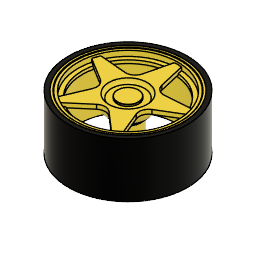
Roda (Autodesk Fusion 360 design; units mm, degrees)
part number: 2026-05-12-10-28-13-651
Autodesk Fusion 360 part; units mm, degrees
sketch "Sketch1" plane through (0, 0, 0) normal (0, 1, 0) x (1, 0, 0)
  circle A0 centre (0, 0) radius 9
  circle A1 centre (0, 0) radius 7.75
  circle A2 centre (0, 0) radius 5
  line L0 (-12.455, -19.928) -> (-2.9617, -11.8295)
  line L1 (12.3158, -20.0143) -> (2.9074, -11.8536)
  arc A3 (2.9074, -11.8536) -> (-2.9617, -11.8295) centre (-0.0412, -15.253) ccw
  line L2 (22.8405, 5.5282) -> (12.1719, -0.8978)
  arc A4 (12.1719, -0.8978) -> (10.3353, -6.4722) centre (14.4937, -4.7526) ccw
  line L3 (15.1038, -18.0035) -> (10.3353, -6.4722)
  line L4 (1.8005, 23.4309) -> (4.6152, 11.2987)
  arc A5 (4.6152, 11.2987) -> (9.3492, 7.8294) centre (8.9988, 12.3157) ccw
  line L5 (21.7896, 8.8012) -> (9.3492, 7.8294)
  line L6 (-21.7278, 8.9529) -> (-9.3195, 7.8808)
  arc A6 (-9.3195, 7.8808) -> (-4.5571, 11.3111) centre (-8.9322, 12.3641) ccw
  line L7 (-1.6371, 23.4429) -> (-4.5571, 11.3111)
  line L8 (-15.229, -17.8977) -> (-10.375, -6.4281)
  arc A7 (-10.375, -6.4281) -> (-12.1657, -0.8388) centre (-14.5192, -4.6743) ccw
  line L9 (-22.8014, 5.6873) -> (-12.1657, -0.8388)
  circle A8 centre (0, 0) radius 25
  circle A9 centre (0, 0) radius 26
  circle A10 centre (0, 0) radius 5.5
  circle A11 centre (0, 0) radius 10.5
  circle A12 centre (0, 0) radius 23.5
  circle A13 centre (0, 0) radius 21.5
  circle A14 centre (0, 0) radius 6.5
  circle A15 centre (0, 0) radius 7
  line L10 (-0.0051, -23.5) -> (-0.0226, -10.753)
  line L11 (22.3482, -7.2668) -> (10.2197, -3.3444)
  line L12 (13.8171, 19.0089) -> (6.3388, 8.6861)
  line L13 (-13.8088, 19.0149) -> (-6.3021, 8.7127)
  line L14 (-22.3514, -7.257) -> (-10.2337, -3.3013)
  circle A16 centre (0, 0) radius 2.9
  line L15 (-2.9, -1.8) -> (2.9, -1.8)
  line L16 (2.9, -1.8) -> (2.9, 1.8)
  line L17 (2.9, 1.8) -> (-2.9, 1.8)
  line L18 (-2.9, 1.8) -> (-2.9, -1.8)
  line L19 (-2.9, -1.8) -> (2.9, 1.8) construction
  line L20 (2.9, -1.8) -> (-2.9, 1.8) construction
  dimension "d7" = 18
  dimension "d8" = 15.5
  dimension "d9" = 10
  dimension "d13" = 4.5
  dimension "d15" = 360
  dimension "d16" = 50
  dimension "d17" = 52
  dimension "d18" = 11
  dimension "d19" = 21
  dimension "d20" = 47
  dimension "d35" = 43
  dimension "d48" = 13
  dimension "d67" = 14
  dimension "d83" = 360
  dimension "d98" = 5.8
  constraint coincident A0.centre A1.centre
  constraint tangent L0 A3
  constraint tangent L1 A3
  constraint concentric A0 A9
  constraint concentric A1 A10
  constraint concentric A1 A11
  constraint concentric A2 A12
  constraint coincident L9.start A12
  constraint coincident L6.start A12
  constraint concentric A2 A13
  constraint concentric A0 A14
  constraint concentric A12 A15
  constraint coincident A12 L10.start
  constraint midpoint A3 L10.end
  constraint concentric A8 A16
  constraint horizontal L15
  constraint perpendicular L15 L16
  constraint parallel L15 L17
  constraint parallel L16 L18
  constraint coincident L19 A0.centre
  constraint coincident L20 A0.centre
  measures "d7" diameter of A0
  measures "d8" diameter of A1
  measures "d9" diameter of A2
  measures "d13" radius of A3
  measures "d16" diameter of A8
  measures "d17" diameter of A9
  measures "d18" diameter of A10
  measures "d19" diameter of A11
  measures "d20" diameter of A12
  measures "d35" diameter of A13
  measures "d48" diameter of A14
  measures "d67" diameter of A15
  measures "d98" diameter of A16
extrude "Extrude1" add sketch "Sketch1" along normal blind 1 contours A2 | A16 L15 L17 | A16 L15 L16 | A16 L16 L17 | A16 L17 | A16 L15 | A16 L17 L18 | A16 L15 L18 makes body 1
extrude "Extrude2" add sketch "Sketch1" along normal blind 2 separate body contours L0 L8 A12 A13 | L0 L1 A3 L2 A4 L3 L4 A5 L5 L6 A6 L7 L8 A7 L9 A13 | L1 L3 A12 A13 | L6 L9 A12 A13 | L4 L7 A12 A13 | L2 L5 A12 A13 | A11 makes body 2
extrude "Extrude3" add sketch "Sketch1" along normal blind 0.2 contours A0 bodies 2
fillet "Fillet1" radius 2.5 1 edges at (-8.3909, 0.2, -3.2545) on bodies 2
extrude "Extrude4" add sketch "Sketch1" against normal blind 2.5 contours A2 | A10 | A16 L15 L17 | A16 L15 L16 | A16 L16 L17 | A16 L17 | A16 L15 | A16 L17 L18 | A16 L15 L18 bodies 1
extrude "Extrude5" add sketch "Sketch1" along normal blind 0.2 contours A1 | A10 | A14 | A15 bodies 1 2
fillet "Fillet2" radius 0.1 1 edges at (-4.6616, 1, 1.8081) on bodies 1
extrude "Extrude6" add sketch "Sketch1" along normal blind 0.5 contours L0 A12 A13 L10 | L8 A12 A13 L14 | L1 A12 A13 L10 | L9 A12 A13 L14 | L3 A12 A13 L11 | L6 A12 A13 L13 | L2 A12 A13 L11 | L7 A12 A13 L13 | L4 A12 A13 L12 | L5 A12 A13 L12 bodies 1
extrude "Extrude7" add sketch "Sketch1" along normal blind 3 contours A8 bodies 1
extrude "Extrude8" add sketch "Sketch1" along normal blind 3.2 contours A9 bodies 1
fillet "Fillet3" radius 0.25 1 edges at (-23.3082, 3, 9.0404) on bodies 1
extrude "Extrude9" add sketch "Sketch1" against normal blind 22.3 contours A8 | A9 bodies 1
extrude "Extrude10" add 1 faces at (-1.4907, -2.5, -0.2732) along direction (0, -1, 0) blind 43 on bodies 1 bodies 1
extrude "Extrude11" add sketch "Sketch1" against normal blind 6 contours A14 bodies 1
extrude "Extrude12" add sketch "Sketch1" against normal blind 3 contours A1 | A15 bodies 1
extrude "Extrude13" add 1 faces at (6.122, -6, 0.5962) along direction (0, -1, 0) blind 3 on bodies 1 bodies 1
extrude "Extrude14" add 1 faces at (7.2803, -3, 0.708) along direction (0, -1, 0) blind 4 on bodies 1 bodies 1
extrude "Extrude15" add sketch "Sketch1" against normal blind 5 contours A0 | A11 bodies 1
fillet "Fillet4" radius 6 1 edges at (-9.7894, -5, -3.797) on bodies 1
extrude "Extrude16" cut 1 faces at (7.2803, -7, 0.708) along direction (0, 1, 0) blind 2 on bodies 1 bodies 1
extrude "Extrude17" cut 1 faces at (6.122, -9, 0.5962) along direction (0, 1, 0) blind 3 on bodies 1 bodies 1
extrude "Extrude18" add 1 faces at (6.122, -6, 0.5962) along direction (0, -1, 0) blind 1 on bodies 1 bodies 1
extrude "Extrude19" add sketch "Sketch1" against normal blind 13 separate body contours A15 makes body 3
extrude "Extrude20" cut 1 faces at (6.7831, -13, 0.6707) along direction (0, 1, 0) blind 9.5 on bodies 3 bodies 1 3
extrude "Extrude21" add 1 faces at (6.7831, -3.5, 0.6707) along direction (0, -1, 0) blind 1.5 on bodies 3 bodies 1 3
fillet "Fillet5" radius 1.5 1 edges at (-7.2255, -5, -2.8025) on bodies 1
fillet "Fillet6" radius 0.5 1 edges at (-6.0601, -7, -2.3505) on bodies 1
extrude "Extrude22" add sketch "Sketch1" against normal blind 2 contours L0 L8 A12 A13 | L0 A12 A13 L10 | L8 A12 A13 L14 | L1 A12 A13 L10 | L9 A12 A13 L14 | L1 L3 A12 A13 | L6 L9 A12 A13 | L3 A12 A13 L11 | L6 A12 A13 L13 | L2 A12 A13 L11 | L7 A12 A13 L13 | L4 L7 A12 A13 | L2 L5 A12 A13 | L4 A12 A13 L12 | L5 A12 A13 L12 bodies 1
extrude "Extrude23" cut 1 faces at (-22.6658, -2, -2.2356) along direction (0, 1, 0) blind 1 on bodies 1 bodies 1
extrude "Extrude24" cut 1 faces at (-1.4907, -45.5, -0.2732) along direction (0, 1, 0) blind 18 on bodies 1 bodies 1
sketch "Sketch2" plane through (0, 0, 0) normal (0, 1, 0) x (1, 0, 0)
  circle A0 centre (0, 0) radius 26
  circle A1 centre (0, 0) radius 28
  dimension "d86" = 52
  dimension "d87" = 56
  constraint coincident A0.centre A1.centre
  constraint concentric A0 A1
  measures "d86" diameter of A0
  measures "d87" diameter of A1
extrude "Extrude25" add sketch "Sketch2" along normal blind 3 separate body makes body 4
extrude "Extrude26" add 1 faces at (27.1323, 0, 2.6828) along direction (0, -1, 0) blind 22 on bodies 4 bodies 4
extrude "Extrude27" add 1 faces at (27.1323, 3, 2.6828) along direction (0, 1, 0) blind 0.3 on bodies 4 bodies 4
extrude "Extrude28" add 1 faces at (27.1323, -22, 2.6828) along direction (0, -1, 0) blind 0.4 on bodies 4 bodies 4
extrude "Extrude29" add 1 faces at (5.7905, -7, 0.5713) along direction (0, -1, 0) blind 20.5 on bodies 1 bodies 1
extrude "Extrude30" cut sketch "Sketch1" against normal blind 48.5 contours A16 L15 L17 | A16 L17 | A16 L15 bodies 1
extrude "Extrude31" add sketch "Sketch1" against normal blind 27 contours A16 L17 | A16 L15 bodies 1
extrude "Extrude32" add sketch "Sketch1" against normal blind 10 contours A16 L15 L17 bodies 1
extrude "Extrude33" add 1 faces at (0.5518, -10, 0.0719) along direction (0, -1, 0) blind 4 on bodies 1 bodies 1
extrude "Extrude34" cut 1 faces at (0.5518, -14, 0.0719) along direction (0, 1, 0) blind 2 on bodies 1 bodies 1
named bodies: "Roda", "Pneu"
